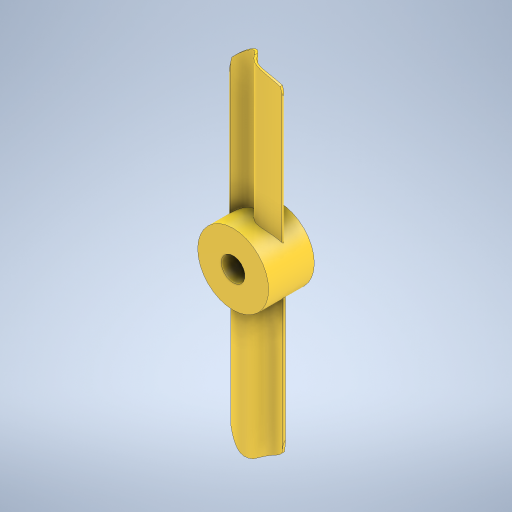
# Autodesk Inventor part: helice
Saved by Autodesk Inventor 2023 (Build 270158000, 158)
## iProperties
Created: 2023-08-09
Part Number: helice
Material: Aço forjado
Document SubType Name: Modeling
Designer: azeve
Density: 7.85 g/cm^3
Appearance: Aço
Author: azeve
Autodesk Inventor part; units mm, degrees
ref_plane "YZ Plane" through (0, 0, 0) normal (1, 0, 0) x (0, 1, 0)
sketch "Esboço1" plane through (0, 0, 0) normal (0, 1, 0) x (-1, 0, 0)
  line L0 (1.5, -1) -> (1.5, -6.8)
  line L1 (0, -9.13) -> (0, 0)
  line L2 (1.5, -1) -> (4.5, -1)
  line L3 (4.5, -1) -> (4.5, -6.8)
  line L4 (4.5, -6.8) -> (1.5, -6.8)
  line L5 (1.5, -6.8) -> (1.5, -1)
  line L6 (4.5, -1) -> (4.5, -3.025)
  line L7 (4.5, -3.025) -> (3.2089, -3.025)
  dimension "d7" = 2.025
  constraints: 16 end point, 2 horizontal, 2 perpendicular, 1 collinear, 1 point on line, 1 vertical
  measures "d7" distance of L2.end L6.end
revolve "Revolução1" add sketch "Esboço1" angle 360 about axis through (0, 0, -9.13) along (0, 0, 1)
sketch "Esboço2" plane through (0, 0, -6.8) normal (0, 0, -1) x (-1, 0, 0)
  point P0 (0, 0)
ref_plane "Plano de trabalho1" through (0, 4.5, 0) normal (0, 1, 0) x (-1, 0, 0)
sketch "Esboço3" plane through (0, 4.5, 0) normal (0, 1, 0) x (-1, 0, 0)
  line L0 (0, -1.0076) -> (0, -3.0576)
  line L1 (1.5, -6.8) -> (-1.5, -6.8) projected
  line L2 (0, -6.8) -> (0, -4.75)
  spline S0 degree 3 poles (-3.2447, -3.9187) (1.3602, -1.0418) (-1.0862, -6.473) (3.2906, -3.9476) knots 0.003297 0.003297 0.003297 0.003297 1 1 1 1
  arc A0 (-3.2447, -3.9187) -> (-3.1074, -4.1385) centre (-3.1988, -4.0428) ccw
  arc A1 (3.4201, -4.172) -> (3.2906, -3.9476) centre (3.3554, -4.0598) ccw
  spline S1 degree 5 poles (-3.1074, -4.1385) (-2.7893, -3.9403) (-2.4619, -3.7491) (-2.1299, -3.5849) (-1.6245, -3.3593) (-1.0853, -3.298) (-0.915, -3.2979) (-0.6047, -3.3915) (-0.3715, -3.6091) (-0.2764, -3.7216) (-0.075, -3.9862) (0.1213, -4.2536) (0.2391, -4.3977) (0.5434, -4.6915) (0.9332, -4.8697) (1.1722, -4.911) (1.7962, -4.9081) (2.3937, -4.7) (2.7428, -4.5432) (3.0868, -4.3646) (3.4201, -4.172) knots 0 0 0 0 0 0 0.251578 0.251578 0.251578 0.36245 0.36245 0.36245 0.461071 0.461071 0.461071 0.584982 0.584982 0.584982 0.741866 0.741866 0.741866 1 1 1 1 1 1
  point P0 (0, 0)
  point P1 (0.5376, -4.3122)
  point P2 (-3.1525, -4.1668)
  dimension "d11" = 2.05
  dimension "d12" = 2.05
  constraints: 5 point on circle, 4 end point, 2 centre point, 2 vertical, 1 midpoint, 10 other
  measures "d11" distance of L0.start L0.end
  measures "d12" distance of L2.start L2.end
ref_plane "Plano de trabalho2" through (0, -4.5, 0) normal (0, 1, 0) x (-1, 0, 0)
sketch "Esboço4" plane through (0, -4.5, 0) normal (0, 1, 0) x (-1, 0, 0)
  spline S0 degree 3 poles (3.2362, -3.929) (-1.3241, -0.9538) (1.058, -6.428) (-3.236, -4.0041) knots 0 0 0 0 1 1 1 1
  arc A0 (3.0364, -4.1503) -> (3.1801, -3.8926) centre (3.1365, -4.0372) ccw
  arc A1 (-3.2021, -4.0231) -> (-3.3421, -4.2822) centre (-3.2884, -4.1439) ccw
  spline S1 degree 5 poles (3.0753, -4.1756) (2.7926, -3.9916) (2.5038, -3.8143) (2.208, -3.6548) (1.7565, -3.4348) (1.2714, -3.3203) (1.1129, -3.2972) (0.8332, -3.3055) (0.5881, -3.4334) (0.5002, -3.5046) (0.3188, -3.6854) (0.1664, -3.8921) (0.0834, -4.0095) (-0.1038, -4.2669) (-0.3153, -4.5039) (-0.4447, -4.6224) (-0.7734, -4.8446) (-1.1611, -4.9447) (-1.3844, -4.9554) (-1.9428, -4.9082) (-2.475, -4.719) (-2.7835, -4.5818) (-3.086, -4.4269) (-3.3808, -4.2605) knots 0 0 0 0 0 0 0.227508 0.227508 0.227508 0.334929 0.334929 0.334929 0.410035 0.410035 0.410035 0.507269 0.507269 0.507269 0.624067 0.624067 0.624067 0.771785 0.771785 0.771785 1 1 1 1 1 1
  point P0 (0, 0)
  point P1 (-3.1444, -4.1909)
  point P2 (3.2362, -3.929)
  point P3 (-0.5415, -4.2978)
  point P4 (-3.2302, -4.0073)
  point P5 (3.0737, -4.1746)
  constraints: 5 point on circle, 2 centre point, 13 other
extrude "Extrusão1" add sketch "Esboço4" along normal blind 2 and the other way blind 20
extrude "Extrusão2" add sketch "Esboço3" along normal blind 20 and the other way blind 2
ref_plane "Plano de trabalho3" through (0, 0, -14.8) normal (0, 0, -1) x (-1, 0, 0)
sketch "Esboço5" plane through (0, 0, -14.8) normal (0, 0, -1) x (-1, 0, 0)
  line L0 (4.9517, 0) -> (-5.7149, 0)
  line L1 (3.1801, -24.5) -> (3.1801, -3.1838) projected
  arc A0 (0.032, -22.1575) -> (3.1801, -20.2125) centre (-1.7722, -15.717) ccw
  line L2 (0.032, -22.1575) -> (0.032, -23.0617)
  arc A1 (-3.1161, -20.2125) -> (0.032, -22.1575) centre (1.8362, -15.717) ccw
  arc A2 (3.1801, 20.2125) -> (0.032, 22.1575) centre (-1.7722, 15.717) ccw
  arc A3 (0.032, 22.1575) -> (-3.1161, 20.2125) centre (1.8362, 15.717) ccw
  line L3 (3.604, -24.9325) -> (-3.9612, -24.9325)
  line L4 (-3.9612, -24.9325) -> (-3.9612, -18.9809)
  line L5 (-3.1161, -20.2125) -> (-3.9612, -16.2534)
  line L6 (-3.9612, -16.2534) -> (-3.9612, -18.9809)
  line L7 (3.604, -24.9325) -> (3.7108, -17.0533)
  line L8 (3.7108, -17.0533) -> (3.1801, -20.2125)
  line L9 (3.604, 24.9325) -> (-3.9612, 24.9325)
  line L10 (-3.9612, 24.9325) -> (-3.9612, 18.9809)
  line L11 (-3.1161, 20.2125) -> (-3.9612, 16.2534)
  line L12 (-3.9612, 16.2534) -> (-3.9612, 18.9809)
  line L13 (3.604, 24.9325) -> (3.7108, 17.0533)
  line L14 (3.7108, 17.0533) -> (3.1801, 20.2125)
  point P0 (0, 0)
  constraints: 28 end point, 12 symmetric about line, 8 point on circle, 4 centre point, 2 horizontal, 1 collinear, 1 perpendicular, 1 point on line, 1 vertical, 3 other
extrude "Extrusão3" cut sketch "Esboço5" along normal mid plane 40
